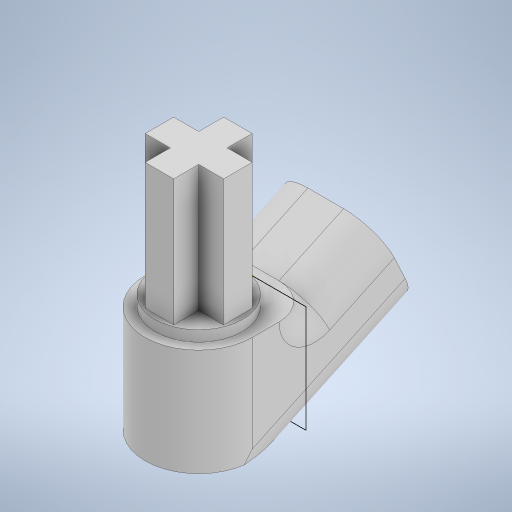
# Autodesk Inventor part: Part4(Part2)
Saved by Autodesk Inventor 2024 (Build 280153000, 153)
## iProperties
Created: 2023-10-11
Part Number: Part4(Part2)
Material: Generic
Document SubType Name: Modeling
Designer: kubad
Density: 1 g/cm^3
Appearance: Default
Author: kubad
## iProperties of the stored document Part4(Part2)_3DPrint.ipt
Created: 2023-10-11
Part Number: Part4(Part2)_3DPrint
Material: Generic
Document SubType Name: Modeling
Designer: kubad
Density: 1 g/cm^3
Appearance: Default
Author: kubad
Autodesk Inventor part; units mm, degrees
ref_plane "YZ Plane" through (0, 0, 0) normal (1, 0, 0) x (0, 1, 0)
ref_plane "XZ Plane" through (0, 0, 0) normal (0, 1, 0) x (-1, 0, 0)
ref_plane "XY Plane" through (0, 0, 0) normal (0, 0, 1) x (1, 0, 0)
sketch "Sketch1" plane through (0, 0, 0) normal (0, 1, 0) x (-1, 0, 0)
  point P0 (0, 0)
sketch "Sketch2" plane through (0, 0, 0) normal (0, 1, 0) x (-1, 0, 0)
  circle A0 centre (0, 0) radius 2.25
  dimension "d0" = 4.5
  constraints: 1 centre point, 1 coincident
  measures "d0" diameter of A0
extrude "Extrusion1" add sketch "Sketch2" along normal blind 7.7
sketch "Sketch3" plane through (0, 7.7, 0) normal (0, 1, 0) x (1, 0, 0)
  circle A0 centre (0, 0) radius 2.45
  dimension "d3" = 4.9
  constraints: 1 centre point, 1 coincident
  measures "d3" diameter of A0
extrude "Extrusion2" add sketch "Sketch3" against normal blind 0.4
sketch "Sketch4" plane through (0, 0, 0) normal (0, -1, 0) x (1, 0, 0)
  circle A0 centre (0, 0) radius 2.45
  constraints: 1 centre point, 1 coincident
extrude "Extrusion3" add sketch "Sketch4" against normal blind 0.6
sketch "Sketch5" plane through (0, 7.7, 0) normal (0, 1, 0) x (1, 0, 0)
  line L0 (0, 0) -> (0, 0.4)
  line L1 (0, 0) -> (0, -0.4)
  circle A0 centre (0, 0) radius 2.45 projected
  line L2 (-2.45, 0) -> (-2.45, -0.4)
  line L3 (2.45, 0) -> (2.45, 0.4)
  line L4 (-2.45, -0.4) -> (2.45, -0.4)
  line L5 (2.45, -0.4) -> (2.45, 0.4)
  line L6 (2.45, 0.4) -> (-2.45, 0.4)
  line L7 (-2.45, 0.4) -> (-2.45, -0.4)
  point P0 (2.4171, 0.4)
  point P1 (2.4171, -0.4)
  point P2 (-2.4171, 0.4)
  point P3 (-2.4171, -0.4)
  dimension "d8" = 0.4
  dimension "d9" = 0.4
  dimension "d10" = 0.4
  dimension "d11" = 0.4
  constraints: 16 end point, 4 vertical, 2 parallel, 2 point on circle, 2 tangent, 1 horizontal, 1 perpendicular
  measures "d8" distance of L0.start L0.end
  measures "d9" distance of L0.start L1.end
  measures "d10" distance of L2.start L2.end
  measures "d11" distance of L3.start L3.end
extrude "Extrusion4" cut sketch "Sketch5" against normal blind 3 contours L0 L6 A0 L4 L1 picked at (0.8057, -0.2667)
extrude "Extrusion5" cut sketch "Sketch5" against normal blind 3 contours L1 L4 A0 L6 L0 picked at (-0.8057, -0.2667)
sketch "Sketch6" plane through (0, 7.7, 0) normal (0, 1, 0) x (1, 0, 0)
  circle A0 centre (0, 0) radius 2
  dimension "d16" = 4
  constraints: 1 centre point, 1 coincident
  measures "d16" diameter of A0
extrude "Extrusion6" cut sketch "Sketch6" against normal blind 5
fillet "Fillet1" radius 0.2 1 edges at (0, 7.3, -2.45)
fillet "Fillet2" radius 0.2 1 edges at (0, 7.7, -2.45)
fillet "Fillet3" radius 0.2 1 edges at (0, 7.3, 2.45)
fillet "Fillet4" radius 0.2 1 edges at (0, 7.7, 2.45)
fillet "Fillet5" radius 0.2 1 edges at (2.0869, 4.7, -0.4)
fillet "Fillet6" radius 0.2 3 edges at (2.0869, 4.7, 0.4) (-2.0869, 4.7, 0.4) (-2.0869, 4.7, -0.4)
fillet "Fillet7" radius 0.2 1 edges at (-2.45, 0.6, 0)
sketch "Sketch7" plane through (0, 0, 0) normal (0, -1, 0) x (1, 0, 0)
  circle A0 centre (0, 0) radius 3
  dimension "d26" = 6
  constraints: 1 centre point, 1 coincident
  measures "d26" diameter of A0
extrude "Extrusion7" add sketch "Sketch7" along normal blind 6
sketch "Sketch8" plane through (0, -6, 0) normal (0, -1, 0) x (1, 0, 0)
  circle A0 centre (0, 0) radius 3 projected
  line L0 (3, -3) -> (-3, -3)
  line L1 (-3, -3) -> (-3, 0)
  line L2 (-3, 0) -> (3, 0)
  line L3 (3, 0) -> (3, -3)
  constraints: 8 end point, 2 parallel, 1 horizontal, 1 horizontal alignment, 1 perpendicular, 1 other
extrude "Extrusion8" add sketch "Sketch8" against normal blind 6 contours L3 L0 A0 | A0 L2 | A0 L0 L1 picked at (0.2225, -0.9749)
sketch "Sketch9" plane through (3, -6, -3) normal (0, 0, -1) x (-1, 0, 0)
  line L0 (0, 0) -> (6, 0) projected
  line L1 (0, 6) -> (6, 6) projected
  line L2 (6, 0) -> (0, 0)
  line L3 (0, 0) -> (0, 6)
  line L4 (0, 6) -> (6, 6)
  line L5 (6, 6) -> (6, 0)
  point P0 (3, 6)
  constraints: 8 end point, 2 parallel, 1 horizontal, 1 perpendicular
sketch "Sketch10" plane through (-3, -6, -3) normal (-1, 0, 0) x (0, 0, 1)
  point P0 (3, 6)
sketch "Sketch11" plane through (3, -6, -3) normal (0, 0, -1) x (-1, 0, 0)
  line L0 (0, 0) -> (6, 0) projected
  line L1 (0, 6) -> (6, 6) projected
  line L2 (0, 0) -> (6, 0)
  line L3 (6, 0) -> (6, 6)
  line L4 (6, 6) -> (0, 6)
  line L5 (0, 6) -> (0, 0)
  point P0 (3, 6)
  constraints: 8 end point, 2 parallel, 1 horizontal, 1 perpendicular
extrude "Extrusion9" add sketch "Sketch11" along normal blind 0.65
sketch "Sketch12" plane through (-3, -6, 0) normal (-1, 0, 0) x (0, 0, 1)
  line L0 (0, 6) -> (-3.65, 6) projected
  line L1 (-3.65, 6) -> (4.05, 6) construction
  line L2 (-3.65, 0) -> (0, 0) projected
  line L3 (-3.65, 0) -> (-9.0947, 5.4447)
  line L4 (-3.65, 0) -> (-3.65, 6)
  line L5 (-9.0947, 5.4447) -> (-6.0947, 8.4447)
  line L6 (-3.65, 6) -> (-6.0947, 8.4447)
  dimension "d35" = 7.7
  constraints: 10 end point, 1 horizontal
  measures "d35" distance of L2.start L3.end
extrude "Extrusion10" add sketch "Sketch12" against normal blind 6
sketch "Sketch13" plane through (3, -0.5553, -9.0947) normal (0, -0.7071068, -0.7071068) x (-1, 0, 0)
  line L0 (0, -7.7) -> (6, -7.7) projected
  line L1 (0, 0) -> (0, -3.4574) projected
  line L2 (6, -7.7) -> (0, -7.7)
  line L3 (0, -7.7) -> (0, 0)
  line L4 (0, 0) -> (6, 0)
  line L5 (6, 0) -> (6, -7.7)
  point P0 (3, -6.0383)
  point P1 (0, -3.4574)
  point P2 (0, -7.7)
  constraints: 8 end point, 2 parallel, 1 horizontal, 1 perpendicular
extrude "Extrusion11" add sketch "Sketch13" along normal blind 1.757
sketch "Sketch14" plane through (-3, -6, 0) normal (-1, 0, 0) x (0, 0, 1)
  line L0 (-10.3371, 4.2023) -> (-4.8924, -1.2424) projected
  line L1 (0, 0) -> (3, 0) projected
  line L2 (-4.8924, -1.2424) -> (3, 0)
  line L3 (-3.65, 0) -> (-4.8924, -1.2424) projected
  line L4 (-4.8924, -1.2424) -> (-3.65, 0)
  line L5 (-3.65, 0) -> (3, 0)
  point P0 (0, 6)
  constraints: 6 end point, 2 collinear
extrude "Extrusion12" add sketch "Sketch14" against normal blind 6
sketch "Sketch15" plane through (0, 0, 0) normal (0, 1, 0) x (1, 0, 0)
  arc A0 (-3, 0) -> (0, -3) centre (0, 0) ccw projected
  circle A1 centre (0, 0) radius 3
  line L0 (-3, 4.8924) -> (-3, -3) projected
  line L1 (-3, -3) -> (0, -3)
  line L2 (0, -3) -> (0, 0)
  line L3 (0, 0) -> (-3, 0)
  line L4 (-3, 0) -> (-3, -3)
  line L5 (3, -3) -> (3, 4.8924) projected
  line L6 (3, -3) -> (0, -3)
  line L7 (0, -3) -> (0, 0)
  line L8 (0, 0) -> (3, 0)
  line L9 (3, 0) -> (3, -3)
  point P0 (0, -3)
  point P1 (0, -3)
  constraints: 16 end point, 4 parallel, 2 horizontal, 2 perpendicular, 1 coincident, 3 other
extrude "Extrusion13" cut sketch "Sketch15" against normal through all contours A0 L1 L0
extrude "Extrusion14" cut sketch "Sketch15" against normal through all contours A1 L5 L6
sketch "Sketch16" plane through (3, 2.4447, -6.0947) normal (0, 0.7071068, -0.7071068) x (-1, 0, 0)
  line L0 (6, -5.9996) -> (0, -5.9996) projected
  line L1 (6, 0) -> (0, 0) projected
  line L2 (6, -5.9996) -> (0, 0)
  line L3 (0, -5.9996) -> (6, 0)
  circle A0 centre (3, -2.9998) radius 1.95
  point P0 (3, 2.5809)
  dimension "d46" = 3.9
  constraints: 4 end point, 1 centre point, 1 midpoint
  measures "d46" diameter of A0
extrude "Extrusion15" cut sketch "Sketch16" against normal blind 6 contours A0 L3 L2 | L2 L3 A0 | A0 L2 L3 | L2 A0 L3
fillet "Fillet8" radius 2 4 edges at (-3, -4.52, -7.6147) (-3, 1.2224, -4.8724) (3, 1.2224, -4.8724) (3, -4.52, -7.6147)
sketch "Sketch17" plane through (0, 7.7, 0) normal (0, 1, 0) x (1, 0, 0)
  circle A0 centre (0, 0) radius 2.45
  constraints: 1 centre point, 1 coincident
extrude "Extrusion16" cut sketch "Sketch17" against normal blind 7.1
sketch "Sketch18" plane through (0, 0.6, 0) normal (0, 1, 0) x (1, 0, 0)
  line L0 (0, 0) -> (0.8, 0)
  line L1 (0, 0) -> (-0.8, 0)
  line L2 (-0.8, 0) -> (0.8, 0)
  line L3 (0.8, 0) -> (0.8, -2.2)
  line L4 (0.8, -2.2) -> (-0.8, -2.2)
  line L5 (-0.8, -2.2) -> (-0.8, 0)
  circle A0 centre (0, 0) radius 2.45
  dimension "d52" = 0.8
  dimension "d53" = 0.8
  dimension "d54" = 2.2
  constraints: 12 end point, 3 horizontal, 2 parallel, 1 centre point, 1 coincident, 1 perpendicular
  measures "d52" distance of L0.start L0.end
  measures "d53" distance of L0.start L1.end
  measures "d54" distance of L2.end L3.end
extrude "Extrusion17" add sketch "Sketch18" against normal blind 1 contours L0 L3 L4 L5 L1 | A0
sketch "Sketch19" plane through (0, 0.6, 0) normal (0, 1, 0) x (1, 0, 0)
  line L0 (0, 0) -> (0.8, 0)
  line L1 (0, 0) -> (-0.8, 0)
  line L2 (-0.8, 0) -> (0.8, 0)
  line L3 (0.8, 0) -> (0.8, -2.2)
  line L4 (0.8, -2.2) -> (-0.8, -2.2)
  line L5 (-0.8, -2.2) -> (-0.8, 0)
  line L6 (-0.8, 0) -> (0.8, 0)
  line L7 (0.8, 0) -> (0.8, 2.2)
  line L8 (0.8, 2.2) -> (-0.8, 2.2)
  line L9 (-0.8, 2.2) -> (-0.8, 0)
  line L10 (0, 0) -> (0, 0.8)
  line L11 (0, 0) -> (0, -0.8)
  line L12 (0, 0.8) -> (2.2, 0.8)
  line L13 (2.2, 0.8) -> (2.2, -0.8)
  line L14 (2.2, -0.8) -> (0, -0.8)
  line L15 (0, -0.8) -> (0, 0.8)
  line L16 (0, 0.8) -> (-2.2, 0.8)
  line L17 (-2.2, 0.8) -> (-2.2, -0.8)
  line L18 (-2.2, -0.8) -> (0, -0.8)
  line L19 (0, -0.8) -> (0, 0.8)
  point P0 (0.8, 0.8)
  point P1 (0.8, -0.8)
  point P2 (-0.8, -0.8)
  point P3 (-0.8, 0.8)
  dimension "d57" = 0.8
  dimension "d58" = 0.8
  dimension "d59" = 2.2
  dimension "d60" = 2.2
  dimension "d61" = 0.8
  dimension "d62" = 0.8
  dimension "d63" = 2.2
  dimension "d64" = 2.2
  constraints: 40 end point, 8 parallel, 6 horizontal, 6 perpendicular
  measures "d57" distance of L0.start L0.end
  measures "d58" distance of L0.start L1.end
  measures "d59" distance of L2.end L3.end
  measures "d60" distance of L7.end L6.end
  measures "d61" distance of L0.start L10.end
  measures "d62" distance of L0.start L11.end
  measures "d63" distance of L13.end L14.end
  measures "d64" distance of L18.end L17.end
extrude "Extrusion18" add sketch "Sketch19" along normal blind 7.1 contours L7 L12 L13 L14 L3
extrude "Extrusion19" add sketch "Sketch19" along normal blind 7.1 contours L14 L3 L4 L5 L18
extrude "Extrusion20" add sketch "Sketch19" along normal blind 7.1 contours L11 L18 L5 L1
extrude "Extrusion21" add sketch "Sketch19" along normal blind 7.1 contours L0 L3 L14 L11
extrude "Extrusion22" add sketch "Sketch19" along normal blind 7.1 contours L1 L9 L16 L10
extrude "Extrusion23" add sketch "Sketch19" along normal blind 7.1 contours L10 L12 L7 L0
extrude "Extrusion24" add sketch "Sketch19" along normal blind 7.1 contours L16 L9 L8 L7 L12
extrude "Extrusion25" add sketch "Sketch19" along normal blind 7.1 contours L5 L18 L17 L16 L9
sketch "Sketch20" plane through (-3, -6.4722, 0) normal (-1, 0, 0) x (0, 0, 1)
  line L0 (0, 6.4722) -> (3, 6.4722) projected
  line L1 (3, 6.4722) -> (-11.0768, 6.4722)
  line L2 (-11.0768, 6.4722) -> (-11.0768, -1.4927)
  line L3 (-11.0768, -1.4927) -> (3, -1.4927)
  line L4 (3, -1.4927) -> (3, 6.4722)
  line L5 (-2.9513, 6.4722) -> (-11.0768, 6.4722)
  line L6 (-11.0768, 6.4722) -> (-11.0768, 9.5471)
  line L7 (-11.0768, 9.5471) -> (-2.9513, 9.5471)
  line L8 (-2.9513, 9.5471) -> (-2.9513, 6.4722)
  constraints: 16 end point, 4 parallel, 2 horizontal, 2 perpendicular, 2 point on line
extrude "Extrusion26" cut sketch "Sketch20" against normal through all contours L0 L4 L3 L2 L1
extrude "Extrusion27" cut sketch "Sketch20" against normal through all contours L1 L6 L7 L8
sketch "Sketch21" plane through (0, 0, 0) normal (0, -1, 0) x (1, 0, 0)
  circle A0 centre (0, 0) radius 3
  line L0 (3, 0) -> (-3, 0)
  dimension "d85" = 6
  constraints: 2 end point, 2 point on circle, 1 centre point, 1 coincident, 1 horizontal
  measures "d85" diameter of A0
extrude "Extrusion28" add sketch "Sketch21" along normal blind 6 contours L0 A0 picked at (0.7485, 0.6631)
sketch "Sketch22" plane through (-2.45, 0, 0) normal (0, 0, -1) x (-1, 0, 0)
  line L0 (-5.45, -6) -> (0.55, -6) projected
  line L1 (0.55, -6) -> (-5.45, -6)
  line L2 (-5.45, -6) -> (-5.45, 0)
  line L3 (-5.45, 0) -> (0.55, 0)
  line L4 (0.55, 0) -> (0.55, -6)
  point P0 (-2.45, 0)
  constraints: 8 end point, 2 parallel, 1 horizontal, 1 perpendicular
extrude "Extrusion29" add sketch "Sketch22" along normal blind 3.5
sketch "Sketch23" plane through (-3, -6, 0) normal (-1, 0, 0) x (0, 0, 1)
  line L0 (-3.5, 6) -> (-13.9764, 10.8852)
  line L1 (-3.5, 6) -> (8.0594, 6) construction
  line L2 (-3.5, 0) -> (-17.595, 6.5726)
  line L3 (-3.5, 0) -> (12.0521, 0) construction
  line L4 (-3.5, 6) -> (-3.5, 0) projected
  line L5 (-3.5, 0) -> (-3.5, 6)
  line L6 (-3.5, 6) -> (-7.1252, 7.6905)
  line L7 (-7.1252, 7.6905) -> (-9.4234, 2.7621)
  point P0 (0, 6)
  dimension "d90" = 155
  dimension "d91" = 155
  dimension "d92" = 4
  constraints: 14 end point, 2 equal length, 2 horizontal, 2 point on line, 1 collinear, 1 perpendicular
  measures "d90" angle of L1 L0
  measures "d91" angle of L3 L2
  measures "d92" distance of L0.start L6.end
extrude "Extrusion30" add sketch "Sketch23" against normal blind 6
sketch "Sketch24" plane through (3, 1.6905, -7.1252) normal (0, 0.4226183, -0.9063078) x (-1, 0, 0)
  line L0 (6, 0) -> (0, 0) projected
  line L1 (6, -3.9587) -> (6, -5.4378) projected
  line L2 (0, 0) -> (6, -5.4378)
  line L3 (6, -5.4378) -> (6, 0)
  line L4 (0, -3.9587) -> (0, -5.4378) projected
  line L5 (6, 0) -> (0, -5.4378)
  circle A0 centre (3, -2.7189) radius 1.95
  point P0 (3, 1.4792)
  dimension "d95" = 3.9
  constraints: 6 end point, 1 centre point, 1 collinear, 1 midpoint
  measures "d95" diameter of A0
extrude "Extrusion31" cut sketch "Sketch24" against normal blind 6 contours A0 L2 L5 | L5 L2 A0 | L2 L5 A0 | L2 A0 L5
fillet "Fillet9" radius 2 1 edges at (-3, -4.6189, -6.4617)
fillet "Fillet10" radius 2 1 edges at (3, -4.6189, -6.4617)
fillet "Fillet11" radius 2 1 edges at (3, 0.8452, -5.3126)
fillet "Fillet12" radius 2 1 edges at (-3, 0.8452, -5.3126)
body "Solid1"
